Autodesk Inventor part; units mm, degrees
(part 2 of 2)
sketch "Sketch7" plane through (0, 0.25, 0) normal (0, 1, 0) x (1, 0, 0)
  circle A0 centre (14, 0) radius 1.65 projected
  circle A1 centre (-14, 0) radius 1.65 projected
  circle A2 centre (32.5, -45) radius 1.65 projected
  circle A3 centre (-32.5, 45) radius 1.65 projected
  circle A4 centre (32.5, 45) radius 1.65 projected
  circle A5 centre (-32.5, -45) radius 1.65 projected
  line L0 (-33, -49.5) -> (33, -49.5) projected
  arc A6 (33, -49.5) -> (38, -44.5) centre (33, -44.5) ccw projected
  line L1 (38, -44.5) -> (38, 44.5) projected
  arc A7 (38, 44.5) -> (33, 49.5) centre (33, 44.5) ccw projected
  line L2 (33, 49.5) -> (-33, 49.5) projected
  arc A8 (-33, 49.5) -> (-38, 44.5) centre (-33, 44.5) ccw projected
  line L3 (-38, 44.5) -> (-38, -44.5) projected
  arc A9 (-38, -44.5) -> (-33, -49.5) centre (-33, -44.5) ccw projected
  line L4 (0.5, -37.05) -> (-0.5, -37.05)
  line L5 (-0.5, -37.05) -> (-0.5, -36.45)
  line L6 (-0.5, -36.45) -> (0.5, -36.45)
  line L7 (0.5, -36.45) -> (0.5, -37.05)
  line L8 (-0.5, -34.95) -> (0.5, -34.95)
  line L9 (0.5, -34.95) -> (0.5, -35.55)
  line L10 (-0.5, -35.55) -> (-0.5, -34.95)
  line L11 (0.5, -35.55) -> (-0.5, -35.55)
  line L12 (-0.5, -33.45) -> (0.5, -33.45)
  line L13 (0.5, -33.45) -> (0.5, -34.05)
  line L14 (-0.5, -34.05) -> (-0.5, -33.45)
  line L15 (0.5, -34.05) -> (-0.5, -34.05)
  line L16 (-0.5, -31.95) -> (0.5, -31.95)
  line L17 (0.5, -31.95) -> (0.5, -32.55)
  line L18 (-0.5, -32.55) -> (-0.5, -31.95)
  line L19 (0.5, -32.55) -> (-0.5, -32.55)
  line L20 (-0.5, -30.45) -> (0.5, -30.45)
  line L21 (0.5, -30.45) -> (0.5, -31.05)
  line L22 (-0.5, -31.05) -> (-0.5, -30.45)
  line L23 (0.5, -31.05) -> (-0.5, -31.05)
  line L24 (-0.5, -28.95) -> (0.5, -28.95)
  line L25 (0.5, -28.95) -> (0.5, -29.55)
  line L26 (-0.5, -29.55) -> (-0.5, -28.95)
  line L27 (0.5, -29.55) -> (-0.5, -29.55)
  line L28 (-0.5, -27.45) -> (0.5, -27.45)
  line L29 (0.5, -27.45) -> (0.5, -28.05)
  line L30 (-0.5, -28.05) -> (-0.5, -27.45)
  line L31 (0.5, -28.05) -> (-0.5, -28.05)
  line L32 (-0.5, -25.95) -> (0.5, -25.95)
  line L33 (0.5, -25.95) -> (0.5, -26.55)
  line L34 (-0.5, -26.55) -> (-0.5, -25.95)
  line L35 (0.5, -26.55) -> (-0.5, -26.55)
  line L36 (-0.5, -24.45) -> (0.5, -24.45)
  line L37 (0.5, -24.45) -> (0.5, -25.05)
  line L38 (-0.5, -25.05) -> (-0.5, -24.45)
  line L39 (0.5, -25.05) -> (-0.5, -25.05)
  line L40 (-0.5, -22.95) -> (0.5, -22.95)
  line L41 (0.5, -22.95) -> (0.5, -23.55)
  line L42 (-0.5, -23.55) -> (-0.5, -22.95)
  line L43 (0.5, -23.55) -> (-0.5, -23.55)
  line L44 (0.5, -30) -> (-0.5, -30) construction
  point P0 (0, 0)
  point P1 (0, -37.05)
  dimension "d71" = 0.6
  dimension "d72" = 1
  dimension "d75" = 1.5
  dimension "d80" = 30
  constraints: 82 end point, 2 horizontal, 2 parallel, 2 point on line, 1 collinear, 1 midpoint, 1 perpendicular, 1 vertical, 1 vertical alignment, 72 other
  measures "d71" distance of L6.end L4.start
  measures "d72" distance of L4.start L4.end
  measures "d75" distance of L6.end L8.end
  measures "d80" distance from line of point (0, 0) L44
extrude "Extrusion6" add sketch "Sketch7" along normal blind 0.035 contours L4 L5 L6 L7 | L8 L9 L11 L10 | L12 L13 L15 L14 | L16 L17 L19 L18 | L20 L21 L23 L22 | L24 L25 L27 L26 | L28 L29 L31 L30 | L32 L33 L35 L34 | L36 L37 L39 L38 | L40 L41 L43 L42
mirror "Mirror1" about plane through (0, 0, 0) normal (0, 0, 1) of "Extrusion6"
equation "\"d54\" = d53"
equation "\"d55\" = d53"
equation "\"d56\" = d53"
equation "\"d57\" = d53"
equation "\"d58\" = d53"
equation "\"d59\" = d53"
equation "\"d65\" = d60"
equation "\"d66\" = d65"
body "Solid1"
